Autodesk Inventor part; units mm, degrees
(part 2 of 2)
  spline S281 degree 2 poles (-34.5157, -46.1095) (-34.4177, -45.9596) (-34.3892, -45.585) (-34.473, -45.3439) knots 0 0 0 1 2 2 2
  spline S282 degree 2 poles (-34.473, -45.3439) (-34.5555, -45.1066) (-34.8129, -44.8229) (-34.9986, -44.733) knots 0 0 0 1 2 2 2
  spline S283 degree 2 poles (-34.9986, -44.733) (-35.1868, -44.6483) (-35.5753, -44.629) (-35.8077, -44.6884) knots 0 0 0 1 2 2 2
  line L180 (-35.8077, -44.6884) -> (-35.157, -46.5598)
  spline S284 degree 2 poles (-36.5684, -49.5827) (-36.7476, -49.1003) (-36.3986, -48.3526) (-35.8023, -48.131) knots 0 0 0 1 2 2 2
  line L181 (-35.8023, -48.131) -> (-33.8538, -47.4072)
  line L182 (-33.8538, -47.4072) -> (-34.0019, -47.0084)
  line L183 (-34.0019, -47.0084) -> (-33.5119, -46.8264)
  line L184 (-33.5119, -46.8264) -> (-33.3638, -47.2252)
  line L185 (-33.3638, -47.2252) -> (-32.3535, -46.8499)
  line L186 (-32.3535, -46.8499) -> (-32.1333, -47.4424)
  line L187 (-32.1333, -47.4424) -> (-33.1437, -47.8177)
  line L188 (-33.1437, -47.8177) -> (-32.7387, -48.9078)
  line L189 (-32.7387, -48.9078) -> (-33.2287, -49.0899)
  line L190 (-33.2287, -49.0899) -> (-33.6337, -47.9998)
  line L191 (-33.6337, -47.9998) -> (-35.3087, -48.622)
  spline S285 degree 2 poles (-35.3087, -48.622) (-35.5746, -48.7207) (-35.86, -48.8484) (-35.9613, -48.9595) knots 0 0 0 1 2 2 2
  spline S286 degree 2 poles (-35.9613, -48.9595) (-36.0517, -49.0536) (-36.073, -49.3338) (-35.9968, -49.5389) knots 0 0 0 1 2 2 2
  spline S287 degree 2 poles (-35.9968, -49.5389) (-35.9432, -49.6833) (-35.7557, -49.9205) (-35.7065, -49.9714) knots 0 0 0 1 2 2 2
  line L192 (-35.7065, -49.9714) -> (-35.6938, -50.0056)
  line L193 (-35.6938, -50.0056) -> (-36.2256, -50.2031)
  spline S288 degree 2 poles (-36.2256, -50.2031) (-36.3332, -50.0529) (-36.5134, -49.7308) (-36.5684, -49.5827) knots 0 0 0 1 2 2 2
  line L194 (-32.4985, -51.3818) -> (-32.5103, -51.3516)
  spline S289 degree 2 poles (-32.5103, -51.3516) (-32.518, -51.2763) (-32.568, -51.1262) (-32.6078, -51.0243) knots 0 0 0 1 2 2 2
  spline S290 degree 2 poles (-32.6078, -51.0243) (-32.7007, -50.7865) (-33.0912, -50.3997) (-33.3776, -50.2681) knots 0 0 0 1 2 2 2
  line L195 (-33.3776, -50.2681) -> (-35.857, -51.2374)
  line L196 (-35.857, -51.2374) -> (-36.0871, -50.6487)
  line L197 (-36.0871, -50.6487) -> (-32.5926, -49.2825)
  line L198 (-32.5926, -49.2825) -> (-32.3625, -49.8712)
  line L199 (-32.3625, -49.8712) -> (-32.8833, -50.0748)
  spline S291 degree 2 poles (-32.8833, -50.0748) (-32.4711, -50.2835) (-32.0497, -50.6713) (-31.9612, -50.8977) knots 0 0 0 1 2 2 2
  spline S292 degree 2 poles (-31.9612, -50.8977) (-31.9258, -50.9882) (-31.8979, -51.0818) (-31.8871, -51.1428) knots 0 0 0 1 2 2 2
  line L200 (-31.8871, -51.1428) -> (-32.4985, -51.3818)
  line L201 (-34.9318, -53.5511) -> (-35.1705, -52.9658)
  line L202 (-35.1705, -52.9658) -> (-31.696, -51.5494)
  line L203 (-31.696, -51.5494) -> (-31.4574, -52.1347)
  line L204 (-31.4574, -52.1347) -> (-34.9318, -53.5511)
  line L205 (-30.8628, -51.9405) -> (-31.1335, -51.2763)
  line L206 (-31.1335, -51.2763) -> (-30.5257, -51.0286)
  line L207 (-30.5257, -51.0286) -> (-30.255, -51.6927)
  line L208 (-30.255, -51.6927) -> (-30.8628, -51.9405)
  line L209 (-32.5597, -59.0185) -> (-32.8183, -58.4417)
  line L210 (-32.8183, -58.4417) -> (-32.4708, -58.2859)
  spline S293 degree 2 poles (-32.4708, -58.2859) (-32.6414, -58.2025) (-32.8771, -58.0729) (-32.9997, -57.968) knots 0 0 0 1 2 2 2
  spline S294 degree 2 poles (-32.9997, -57.968) (-33.1135, -57.8725) (-33.2941, -57.6381) (-33.372, -57.4644) knots 0 0 0 1 2 2 2
  spline S295 degree 2 poles (-33.372, -57.4644) (-33.498, -57.1834) (-33.4772, -56.6057) (-33.3263, -56.3382) knots 0 0 0 1 2 2 2
  spline S296 degree 2 poles (-33.3263, -56.3382) (-33.1753, -56.0707) (-32.5927, -55.5875) (-32.1601, -55.3935) knots 0 0 0 1 2 2 2
  spline S297 degree 2 poles (-32.1601, -55.3935) (-31.7091, -55.1913) (-30.9465, -55.1292) (-30.6076, -55.2214) knots 0 0 0 1 2 2 2
  spline S298 degree 2 poles (-30.6076, -55.2214) (-30.3012, -55.3105) (-29.8091, -55.7249) (-29.6781, -56.017) knots 0 0 0 1 2 2 2
  spline S299 degree 2 poles (-29.6781, -56.017) (-29.5638, -56.2721) (-29.5076, -56.7043) (-29.5315, -56.9681) knots 0 0 0 1 2 2 2
  line L211 (-29.5315, -56.9681) -> (-28.0526, -56.305)
  line L212 (-28.0526, -56.305) -> (-27.794, -56.8818)
  line L213 (-27.794, -56.8818) -> (-32.5597, -59.0185)
  line L214 (-31.9864, -58.0688) -> (-30.0084, -57.1819)
  spline S300 degree 2 poles (-30.0084, -57.1819) (-30.001, -56.9211) (-30.0759, -56.5461) (-30.1637, -56.3501) knots 0 0 0 1 2 2 2
  spline S301 degree 2 poles (-30.1637, -56.3501) (-30.3627, -55.9065) (-31.2536, -55.702) (-31.8821, -55.9838) knots 0 0 0 1 2 2 2
  spline S302 degree 2 poles (-31.8821, -55.9838) (-32.4885, -56.2557) (-32.9557, -56.927) (-32.7651, -57.3521) knots 0 0 0 1 2 2 2
  spline S303 degree 2 poles (-32.7651, -57.3521) (-32.664, -57.5777) (-32.2514, -57.9433) (-31.9864, -58.0688) knots 0 0 0 1 2 2 2
  line L215 (-31.8928, -60.4287) -> (-32.1623, -59.8569)
  line L216 (-32.1623, -59.8569) -> (-28.7686, -58.2568)
  line L217 (-28.7686, -58.2568) -> (-28.499, -58.8285)
  line L218 (-28.499, -58.8285) -> (-31.8928, -60.4287)
  line L219 (-27.9156, -58.6027) -> (-28.2215, -57.954)
  line L220 (-28.2215, -57.954) -> (-27.6278, -57.6741)
  line L221 (-27.6278, -57.6741) -> (-27.3219, -58.3228)
  line L222 (-27.3219, -58.3228) -> (-27.9156, -58.6027)
  spline S304 degree 2 poles (-31.1287, -62.2156) (-31.295, -61.8775) (-31.4011, -61.2027) (-31.3941, -60.9599) knots 0 0 0 1 2 2 2
  line L223 (-31.3941, -60.9599) -> (-30.7578, -60.647)
  line L224 (-30.7578, -60.647) -> (-30.7435, -60.6761)
  spline S305 degree 2 poles (-30.7435, -60.6761) (-30.7659, -60.7774) (-30.8075, -61.0417) (-30.8034, -61.2429) knots 0 0 0 1 2 2 2
  spline S306 degree 2 poles (-30.8034, -61.2429) (-30.8028, -61.4186) (-30.7329, -61.8178) (-30.6417, -62.0032) knots 0 0 0 1 2 2 2
  spline S307 degree 2 poles (-30.6417, -62.0032) (-30.5755, -62.1377) (-30.3617, -62.4164) (-30.2751, -62.464) knots 0 0 0 1 2 2 2
  spline S308 degree 2 poles (-30.2751, -62.464) (-30.1541, -62.5355) (-29.9513, -62.5531) (-29.7913, -62.4745) knots 0 0 0 1 2 2 2
  spline S309 degree 2 poles (-29.7913, -62.4745) (-29.5913, -62.3761) (-29.4914, -62.056) (-29.56, -61.7421) knots 0 0 0 1 2 2 2
  spline S310 degree 2 poles (-29.56, -61.7421) (-29.5882, -61.6205) (-29.6871, -61.2357) (-29.7204, -61.0669) knots 0 0 0 1 2 2 2
  spline S311 degree 2 poles (-29.7204, -61.0669) (-29.7973, -60.6261) (-29.5036, -60.0482) (-29.1727, -59.8854) knots 0 0 0 1 2 2 2
  spline S312 degree 2 poles (-29.1727, -59.8854) (-28.7146, -59.6601) (-27.8058, -60.0665) (-27.5268, -60.6337) knots 0 0 0 1 2 2 2
  spline S313 degree 2 poles (-27.5268, -60.6337) (-27.3891, -60.9137) (-27.2483, -61.5489) (-27.259, -61.7934) knots 0 0 0 1 2 2 2
  line L225 (-27.259, -61.7934) -> (-27.8662, -62.0921)
  line L226 (-27.8662, -62.0921) -> (-27.8805, -62.063)
  spline S314 degree 2 poles (-27.8805, -62.063) (-27.8132, -61.759) (-27.8743, -61.1298) (-28.0085, -60.8571) knots 0 0 0 1 2 2 2
  spline S315 degree 2 poles (-28.0085, -60.8571) (-28.1462, -60.5771) (-28.572, -60.308) (-28.8084, -60.4242) knots 0 0 0 1 2 2 2
  spline S316 degree 2 poles (-28.8084, -60.4242) (-29.0229, -60.5297) (-29.1175, -60.8607) (-29.0578, -61.1474) knots 0 0 0 1 2 2 2
  spline S317 degree 2 poles (-29.0578, -61.1474) (-29.0297, -61.2871) (-28.9413, -61.632) (-28.8973, -61.8225) knots 0 0 0 1 2 2 2
  spline S318 degree 2 poles (-28.8973, -61.8225) (-28.8094, -62.2399) (-29.0561, -62.8308) (-29.4306, -63.015) knots 0 0 0 1 2 2 2
  spline S319 degree 2 poles (-29.4306, -63.015) (-29.6488, -63.1223) (-30.1182, -63.141) (-30.3423, -63.0435) knots 0 0 0 1 2 2 2
  spline S320 degree 2 poles (-30.3423, -63.0435) (-30.579, -62.9386) (-30.9588, -62.561) (-31.1287, -62.2156) knots 0 0 0 1 2 2 2
  line L227 (-28.7718, -66.6273) -> (-29.0646, -66.0671)
  line L228 (-29.0646, -66.0671) -> (-27.1685, -65.0761)
  spline S321 degree 2 poles (-27.1685, -65.0761) (-26.9387, -64.956) (-26.5662, -64.7065) (-26.4815, -64.5799) knots 0 0 0 1 2 2 2
  spline S322 degree 2 poles (-26.4815, -64.5799) (-26.3915, -64.446) (-26.397, -64.138) (-26.5059, -63.9297) knots 0 0 0 1 2 2 2
  spline S323 degree 2 poles (-26.5059, -63.9297) (-26.6148, -63.7214) (-27.0683, -63.3961) (-27.3586, -63.2781) knots 0 0 0 1 2 2 2
  line L229 (-27.3586, -63.2781) -> (-29.8435, -64.5769)
  line L230 (-29.8435, -64.5769) -> (-30.1363, -64.0167)
  line L231 (-30.1363, -64.0167) -> (-25.5076, -61.5974)
  line L232 (-25.5076, -61.5974) -> (-25.2148, -62.1576)
  line L233 (-25.2148, -62.1576) -> (-26.8881, -63.0322)
  spline S324 degree 2 poles (-26.8881, -63.0322) (-26.5305, -63.1653) (-26.0401, -63.5262) (-25.8975, -63.7991) knots 0 0 0 1 2 2 2
  spline S325 degree 2 poles (-25.8975, -63.7991) (-25.6422, -64.2875) (-25.9996, -65.1783) (-26.6136, -65.4993) knots 0 0 0 1 2 2 2
  line L234 (-26.6136, -65.4993) -> (-28.7718, -66.6273)
  point P0 (0, 0)
  constraints: 2 point on circle, 1 centre point, 1 other
extrude "Extrusion3" add sketch "Skizze3" along normal blind 1
